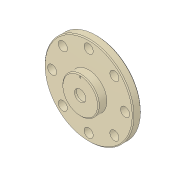
# Autodesk Inventor part: XM430_HORN
Saved by Autodesk Inventor 2019.4 (Build 234330000, 330)
## iProperties
Created: 2019-10-21
Part Number: XM430_HORN
Material: 一般
Document SubType Name: Modeling
Designer: y6tada
Density: 1 g/cm^3
Appearance: 淡いベージュ
Author: y6tada
Autodesk Inventor part; units mm, degrees
ref_plane "YZ Plane" through (0, 0, 0) normal (1, 0, 0) x (0, 1, 0)
ref_plane "XZ Plane" through (0, 0, 0) normal (0, 1, 0) x (-1, 0, 0)
ref_plane "XY Plane" through (0, 0, 0) normal (0, 0, 1) x (1, 0, 0)
sketch "スケッチ1" plane through (0, 0, 0) normal (1, 0, 0) x (0, 1, 0)
  line L0 (0, 0) -> (0, 10.078026) construction
  line L1 (4, 0) -> (4, -0.45)
  line L2 (4, -0.45) -> (3, -0.45)
  line L3 (3, -0.45) -> (3, 3.4)
  line L4 (3, 3.4) -> (1.25, 3.4)
  line L5 (1.25, 3.4) -> (1.25, 3.85)
  line L6 (1.25, 3.85) -> (4, 3.85)
  line L7 (4, 3.85) -> (4, 2)
  line L8 (4, 2) -> (9.75, 2)
  line L9 (9.75, 2) -> (9.75, 0.2)
  line L10 (9.75, 0.2) -> (9, 0.2)
  line L11 (9, 0.2) -> (9, 0)
  line L12 (9, 0) -> (4, 0)
  line L13 (4, 2) -> (4, 0) construction
  dimension "d0" = 19.5
  dimension "d1" = 18
  dimension "d2" = 2
  dimension "d3" = 1.8
  dimension "d4" = 8
  dimension "d5" = 4.3
  dimension "d6" = 2.5
  dimension "d7" = 1.85
  dimension "d8" = 6
  dimension "d10" = 3.85
  dimension "d37" = 3.4
  constraints: 28 end point, 10 perpendicular, 3 vertical, 1 horizontal, 1 point on line
  measures "d0" diameter of L9 L0
  measures "d1" diameter of L11 L0
  measures "d2" distance between parallel lines of L12 L8
  measures "d3" distance of L8.end L9.end
  measures "d4" diameter of L7 L0
  measures "d5" distance between parallel lines of L2 L6
  measures "d6" diameter of L5 L0
  measures "d7" distance between parallel lines of L6 L8
  measures "d8" diameter of L3 L0
  measures "d10" distance of L2.end L3.end
  measures "d37" distance between parallel lines of L4 L12
revolve "回転1" add sketch "スケッチ1" angle 360 about axis through (0, 0, 0) along (0, 0, 1)
sketch "スケッチ2" plane through (0, 0, 2) normal (0, 0, 1) x (1, 0, 0)
  circle A0 centre (0, 0) radius 8 construction
  line L0 (0, 8) -> (0, 0) construction
  point P0 (-5.656854, 5.656854)
  point P1 (-8, 0)
  point P2 (-5.656854, -5.656854)
  point P3 (0, -8)
  point P4 (5.656854, -5.656854)
  point P5 (8, 0)
  point P6 (5.656854, 5.656854)
  dimension "d13" = 16
  dimension "d16" = 360
  constraints: 2 end point, 1 coincident, 1 vertical, 1 vertical alignment, 11 other
hole "穴1" at (0, 8, 2) at (-5.656854, 5.656854, 2) at (-8, 0, 2) at (-5.656854, -5.656854, 2) at (0, -8, 2) at (5.656854, -5.656854, 2) at (8, 0, 2) at (5.656854, 5.656854, 2) direction (0, 0, -1) diameter 2 end through all
chamfer "面取り1" distance 0.2 angle 45 3 edges at (0, -9.75, 2) (0, -9.75, 0.2) (0, -4, 3.85)
sketch "スケッチ3" plane through (0, 0, 3.85) normal (0, 0, 1) x (1, 0, 0)
  line L0 (0, 3.5) -> (0, 0) construction
  dimension "d29" = 3.5
  constraints: 2 end point, 1 coincident, 1 vertical
  measures "d29" distance of L0.start L0.end
hole "穴2" at (0, 3.5, 3.85) direction (0, 0, -1) diameter 0.35 depth 0.2 tip angle 118
